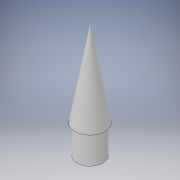
# Autodesk Inventor part: NoseCone_Mk III
Saved by Autodesk Inventor 2017 (Build 210142000, 142)
## iProperties
Created: 2017-05-23
Part Number: NoseCone_Mk III
Material: Generic
Document SubType Name: Modeling
Designer: Harrison
Density: 1 g/cm^3
Appearance: Default
Author: Harrison
Autodesk Inventor part; units mm, degrees
ref_plane "YZ Plane" through (0, 0, 0) normal (1, 0, 0) x (0, 1, 0)
ref_plane "XZ Plane" through (0, 0, 0) normal (0, 1, 0) x (-1, 0, 0)
ref_plane "XY Plane" through (0, 0, 0) normal (0, 0, 1) x (1, 0, 0)
sketch "Sketch1" plane through (0, 0, 0) normal (0, 0, 1) x (1, 0, 0)
  line L0 (0, 0) -> (0, 76.2)
  line L1 (11.6078, 0) -> (76.2, 0) construction
  line L2 (11.6078, 0) -> (13.462, 0)
  line L3 (11.6078, 0) -> (13.462, 0) construction
  line L4 (13.462, 0) -> (0, 76.2)
  line L5 (11.6078, 0) -> (11.6078, -25.4)
  line L6 (11.6078, -25.4) -> (0, -25.4)
  line L7 (0, -25.4) -> (0, 0)
  line L8 (10.3378, 1.27) -> (11.948, 1.27)
  line L9 (11.948, 1.27) -> (1.27, 61.7113)
  line L10 (10.3378, -24.13) -> (10.3378, -1.27)
  line L11 (10.3378, -1.27) -> (10.3378, 1.27)
  line L12 (10.3378, -24.13) -> (10.3378, -25.4)
  line L13 (1.27, 61.7113) -> (0, 68.9)
  dimension "d0" = 76.2
  dimension "d1" = 90
  dimension "d2" = 13.462
  dimension "d3" = 0
  dimension "d4" = 11.6078
  dimension "d5" = 25.4
  dimension "d6" = 1.27
  dimension "d7" = 1.27
  constraints: 28 end point, 3 horizontal, 3 perpendicular, 2 point on line, 2 vertical, 1 collinear
  measures "d0" distance of L0.start L0.end
  measures "d1" angle of L1 L0
  measures "d2" distance of L0.start L2.end
  measures "d3" distance between parallel lines of L2 L3
  measures "d4" distance of L1.start L0.start
  measures "d5" distance of L1.start L5.end
  measures "d6" distance between parallel lines of L4 L9
  measures "d7" distance between parallel lines of L5 L10
revolve "Revolution1" add sketch "Sketch1" angle 360 about axis through (0, 0, 0) along (0, 1, 0) contours L0 L4 L2 L5 L6 L12 L10 L11 L8 L9 L13
sketch "Sketch2" plane through (0, -25.4, 0) normal (0, -1, 0) x (1, 0, 0)
  circle A0 centre (0, 0) radius 10.3378 projected
  line L0 (10.337, -0.127) -> (8.0518, -0.127)
  line L1 (10.337, -0.127) -> (8.0518, -0.127)
  line L2 (10.337, 0.127) -> (8.0518, 0.127)
  line L3 (8.0518, 1.27) -> (8.0518, 0.127)
  line L4 (8.0518, -0.127) -> (8.0518, -1.27)
  line L5 (8.0518, -1.27) -> (7.7978, -1.27)
  line L6 (8.0518, 1.27) -> (7.7978, 1.27)
  line L7 (7.7978, 1.27) -> (7.7978, -1.27)
  constraints: 16 end point, 2 horizontal, 2 point on circle, 1 vertical
extrude "Extrusion1" add sketch "Sketch2" against normal blind 1.27 contours A0 L0 L4 L5 L7 L6 L3 L2 picked at (7.8825, -0.0423)
body "Solid1"
